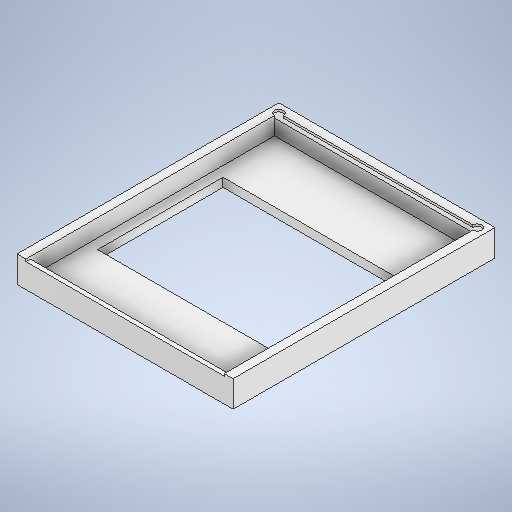
# Autodesk Inventor part: Module Cover
Saved by Autodesk Inventor 2025 (Build 290162000, 162)
## iProperties
Created: 2023-10-04
Part Number: Module Cover
Material: ABS Plastic
Document SubType Name: Modeling
Designer: cfang
Density: 1.06 g/cm^3
Appearance: Smooth - White
Author: cfang
Autodesk Inventor part; units mm, degrees
ref_plane "YZ Plane" through (0, 0, 0) normal (1, 0, 0) x (0, 1, 0)
ref_plane "XZ Plane" through (0, 0, 0) normal (0, 1, 0) x (-1, 0, 0)
ref_plane "XY Plane" through (0, 0, 0) normal (0, 0, 1) x (1, 0, 0)
sketch "Sketch1" plane through (0, 0, 0) normal (0, 1, 0) x (-1, 0, 0)
  line L0 (-24.55, -31.25) -> (24.55, -31.25)
  line L1 (24.55, -31.25) -> (24.55, 31.25)
  line L2 (24.55, 31.25) -> (-24.55, 31.25)
  line L3 (-24.55, 31.25) -> (-24.55, -31.25)
  line L4 (-24.55, -31.25) -> (24.55, 31.25) construction
  line L5 (24.55, -31.25) -> (-24.55, 31.25) construction
  point P0 (0, 0)
  dimension "d0" = 62.5
  dimension "d1" = 49.1
  constraints: 12 end point, 2 midpoint, 2 parallel, 1 horizontal, 1 perpendicular
  measures "d0" distance of L0.end L1.end
  measures "d1" distance of L1.end L2.end
extrude "Extrusion1" add sketch "Sketch1" along normal blind 6
sketch "Sketch2" plane through (0, 6, 0) normal (0, 1, 0) x (1, 0, 0)
  line L0 (22.55, 29.25) -> (-22.55, 29.25)
  line L1 (-22.55, 29.25) -> (-22.55, -29.25)
  line L2 (-22.55, -29.25) -> (22.55, -29.25)
  line L3 (22.55, -29.25) -> (22.55, 29.25)
  line L4 (22.55, 29.25) -> (-22.55, -29.25) construction
  line L5 (-22.55, 29.25) -> (22.55, -29.25) construction
  line L6 (-24.55, 31.25) -> (-24.55, -31.25) projected
  line L7 (-24.55, -31.25) -> (24.55, -31.25) projected
  arc A0 (-22.55, -28.25) -> (-21.55, -29.25) centre (-22.55, -29.25) ccw
  arc A1 (21.55, -29.25) -> (22.55, -28.25) centre (22.55, -29.25) ccw
  arc A2 (-21.55, 29.25) -> (-22.55, 28.25) centre (-22.55, 29.25) ccw
  arc A3 (22.55, 28.25) -> (21.55, 29.25) centre (22.55, 29.25) ccw
  point P0 (0, 0)
  dimension "d4" = 2
  dimension "d5" = 2
  dimension "d32" = 1
  dimension "d33" = 1
  dimension "d34" = 1
  dimension "d35" = 1
  constraints: 12 end point, 8 point on circle, 8 point on line, 4 centre point, 4 coincident, 2 midpoint, 2 parallel, 1 horizontal, 1 perpendicular
  measures "d4" distance between parallel lines of L6 L1
  measures "d5" distance between parallel lines of L7 L2
  measures "d32" radius of A0
  measures "d33" radius of A1
  measures "d34" radius of A2
  measures "d35" radius of A3
extrude "Extrusion2" cut sketch "Sketch2" against normal blind 0.5
sketch "Sketch3" plane through (0, 5.5, 0) normal (0, 1, 0) x (1, 0, 0)
  line L0 (-22.55, -28.25) -> (-22.55, 28.25) projected
  line L1 (22.55, 28.25) -> (-22.55, 28.25)
  line L2 (-22.55, 28.25) -> (-22.55, -28.25)
  line L3 (-22.55, -28.25) -> (22.55, -28.25)
  line L4 (22.55, -28.25) -> (22.55, 28.25)
  line L5 (22.55, 28.25) -> (-22.55, -28.25) construction
  line L6 (-22.55, 28.25) -> (22.55, -28.25) construction
  line L7 (21.55, -29.25) -> (-21.55, -29.25) projected
  point P0 (0, 0)
  point P1 (-22.3, -29)
  point P2 (-22.3, 29)
  point P3 (22.3, -29)
  point P4 (-22.3, 28)
  point P5 (-21.55, -29.25)
  dimension "d8" = 1
  constraints: 12 end point, 2 midpoint, 2 parallel, 1 horizontal, 1 perpendicular, 3 other
extrude "Extrusion3" cut sketch "Sketch3" against normal blind 3.5
sketch "Sketch8" plane through (0, 2, 0) normal (0, 1, 0) x (1, 0, 0)
  line L0 (-20.25, -14.25) -> (20.25, -14.25)
  line L1 (20.25, -14.25) -> (20.25, 14.25)
  line L2 (20.25, 14.25) -> (-20.25, 14.25)
  line L3 (-20.25, 14.25) -> (-20.25, -14.25)
  line L4 (-20.25, -14.25) -> (20.25, 14.25) construction
  line L5 (20.25, -14.25) -> (-20.25, 14.25) construction
  point P0 (0, 0)
  dimension "d28" = 28.5
  dimension "d29" = 40.5
  constraints: 12 end point, 2 midpoint, 2 parallel, 1 horizontal, 1 perpendicular
  measures "d28" distance of L0.end L1.end
  measures "d29" distance of L1.end L2.end
extrude "Extrusion6" cut sketch "Sketch8" against normal through all
sketch "Sketch9" plane through (0, 6, 0) normal (0, 1, 0) x (1, 0, 0)
  line L0 (24.55, -28.25) -> (-24.55, -28.25)
  line L1 (-24.55, -28.25) -> (-24.55, -31.25)
  line L2 (-24.55, -31.25) -> (24.55, -31.25)
  line L3 (24.55, -31.25) -> (24.55, -28.25)
  line L4 (24.55, -31.25) -> (24.55, 31.25) projected
  line L5 (-21.55, 29.25) -> (21.55, 29.25) projected
  point P0 (0, 0)
  dimension "d36" = 57.5
  constraints: 8 end point, 2 parallel, 1 horizontal, 1 perpendicular, 1 point on line
  measures "d36" distance between parallel lines of L0 L5
extrude "Extrusion7" cut sketch "Sketch9" against normal through all
sketch "Sketch10" plane through (0, 2, 0) normal (0, 1, 0) x (1, 0, 0)
  line L0 (22.55, -28.25) -> (-22.55, -28.25) projected
  line L1 (-22.55, -28.25) -> (22.55, -28.25)
  line L2 (22.55, -28.25) -> (22.55, -27.25)
  line L3 (22.55, -27.25) -> (-22.55, -27.25)
  line L4 (-22.55, -27.25) -> (-22.55, -28.25)
  point P0 (0, 0)
  dimension "d39" = 1
  constraints: 8 end point, 2 parallel, 1 horizontal, 1 perpendicular
  measures "d39" distance between parallel lines of L0 L3
extrude "Extrusion8" add sketch "Sketch10" along normal up to surface (3.5 mm away)
equation "\"d5\" = d4"
equation "\"d33\" = d32"
equation "\"d34\" = d32"
equation "\"d35\" = d32"
body "Solid1"
